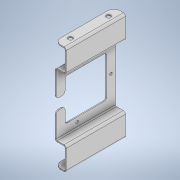
# Autodesk Inventor part: LiDAR_LD19_LD_Plate_1mm_60mmW_Hole
Saved by Autodesk Inventor 2022 (Build 260153000, 153)
## iProperties
Created: 2023-09-22
Part Number: LiDAR_LD19_LD_Plate_1mm_60mmW_Hole
Material: 一般
Document SubType Name: Sheet Metal
Designer: gisen-neige2
Density: 1 g/cm^3
Sheet Metal Rule: Default_mm
Appearance: 既定
Author: gisen-neige2
Autodesk Inventor part; units mm, degrees
ref_plane "YZ Plane" through (0, 0, 0) normal (1, 0, 0) x (0, 1, 0)
ref_plane "XZ Plane" through (0, 0, 0) normal (0, 1, 0) x (-1, 0, 0)
sketch "スケッチ1" plane through (0, 0, 0) normal (0, 1, 0) x (-1, 0, 0)
  line L0 (5.5, 28) -> (-5.5, 28)
  line L1 (-5.5, 28) -> (-5.5, -28)
  line L2 (-5.5, -28) -> (5.5, -28)
  line L3 (5.5, -28) -> (5.5, 28)
  line L4 (5.5, 28) -> (-5.5, -28) construction
  line L5 (-5.5, 28) -> (5.5, -28) construction
  point P0 (0, 0)
  dimension "d0" = 11
  dimension "d1" = 56
  measures "d0" distance of L2.end L1.end
  measures "d1" distance of L1.end L0.end
extrude "プレート1" add sketch "スケッチ1" along normal blind 1
sketch "スケッチ2" plane through (4.5, 1, 28) normal (1, 0, 0) x (0, 1, 0)
  line L0 (0, -56) -> (0, 0)
  line L1 (0, 0) -> (-22, 0)
  line L2 (-22, 0) -> (-22, -56)
  line L3 (-22, -56) -> (0, -56)
  constraints: 6 end point, 1 horizontal, 1 perpendicular, 1 vertical
edge flange "フランジ1" height 22 angle 90 thickness 1 bend radius 1 thickness toward (1, 0, 0) relief tear relief width 1 relief depth 0.5 edges at (5.5, 0, 0) wall of the first edge with corners at (4.5, 1, -28) (4.5, 1, 28) (4.5, -21, 28) (4.5, -21, -28)
bend "曲げ1"
corner "コーナー1"
sketch "スケッチ3" plane through (5.5, -20, 28) normal (0, -1, 0) x (1, 0, 0)
  line L0 (0, -56) -> (0, 0)
  line L1 (0, 0) -> (-10.5, 0)
  line L2 (-10.5, 0) -> (-10.5, -56)
  line L3 (-10.5, -56) -> (0, -56)
  constraints: 6 end point, 1 horizontal, 1 perpendicular, 1 vertical
edge flange "フランジ2" height 10.5 angle 90 thickness 1 bend radius 1 thickness toward (0, -1, 0) relief tear relief width 1 relief depth 0.5 edges at (4.5, -21, 0) wall of the first edge with corners at (5.5, -20, -28) (5.5, -20, 28) (-5, -20, 28) (-5, -20, -28)
bend "曲げ2"
corner "コーナー2"
sketch "スケッチ4" plane through (-4, -20, -28) normal (-1, 0, 0) x (0, -1, 0)
  line L0 (0, 56) -> (0, 0)
  line L1 (0, 0) -> (60, 0)
  line L2 (60, 0) -> (60, 56)
  line L3 (60, 56) -> (0, 56)
  constraints: 6 end point, 1 horizontal, 1 perpendicular, 1 vertical
edge flange "フランジ3" height 60 angle 90 thickness 1 bend radius 1 thickness toward (-1, 0, 0) relief tear relief width 1 relief depth 0.5 edges at (-5, -21, 0) wall of the first edge with corners at (-4, -20, 28) (-4, -20, -28) (-4, -80, -28) (-4, -80, 28)
bend "曲げ3"
corner "コーナー3"
sketch "スケッチ5" plane through (-5, -79, -28) normal (0, -1, 0) x (1, 0, 0)
  line L0 (0, 56) -> (0, 0)
  line L1 (0, 0) -> (10.5, 0)
  line L2 (10.5, 0) -> (10.5, 56)
  line L3 (10.5, 56) -> (0, 56)
  constraints: 6 end point, 1 horizontal, 1 perpendicular, 1 vertical
edge flange "フランジ4" height 10.5 angle 90 thickness 1 bend radius 1 thickness toward (0, -1, 0) relief tear relief width 1 relief depth 0.5 edges at (-4, -80, 0) wall of the first edge with corners at (-5, -79, 28) (-5, -79, -28) (5.5, -79, -28) (5.5, -79, 28)
bend "曲げ4"
corner "コーナー4"
sketch "スケッチ6" plane through (4.5, -79, 28) normal (1, 0, 0) x (0, 1, 0)
  line L0 (0, -56) -> (0, 0)
  line L1 (0, 0) -> (-22, 0)
  line L2 (-22, 0) -> (-22, -56)
  line L3 (-22, -56) -> (0, -56)
  constraints: 6 end point, 1 horizontal, 1 perpendicular, 1 vertical
edge flange "フランジ5" height 22 angle 90 thickness 1 bend radius 1 thickness toward (1, 0, 0) relief tear relief width 1 relief depth 0.5 edges at (5.5, -80, 0) wall of the first edge with corners at (4.5, -79, -28) (4.5, -79, 28) (4.5, -101, 28) (4.5, -101, -28)
bend "曲げ5"
corner "コーナー5"
sketch "スケッチ7" plane through (5.5, -100, 28) normal (0, -1, 0) x (1, 0, 0)
  line L0 (0, -56) -> (0, 0)
  line L1 (0, 0) -> (-11, 0)
  line L2 (-11, 0) -> (-11, -56)
  line L3 (-11, -56) -> (0, -56)
  constraints: 6 end point, 1 horizontal, 1 perpendicular, 1 vertical
edge flange "フランジ6" height 11 angle 90 thickness 1 bend radius 1 thickness toward (0, -1, 0) relief tear relief width 1 relief depth 0.5 edges at (4.5, -101, 0) wall of the first edge with corners at (5.5, -100, -28) (5.5, -100, 28) (-5.5, -100, 28) (-5.5, -100, -28)
bend "曲げ6"
corner "コーナー6"
fillet "コーナーR1" radius 6 4 edges at (-5.5, -100.5, 28) (-5.5, 0.5, -28) (-5.5, 0.5, 28) (-5.5, -100.5, -28)
sketch "スケッチ8" plane through (-4, -22, 28) normal (1, 0, 0) x (0, 0, -1)
  circle A0 centre (19.77, -51.9851) radius 3.6
  circle A1 centre (19.77, -5.1851) radius 3.6
  circle A2 centre (51.69, -28.5851) radius 3.6
  line L0 (9, -47.5851) -> (9, -9.5851)
  circle A3 centre (19.77, -51.9851) radius 2.23
  circle A4 centre (19.77, -5.1851) radius 2.23
  circle A5 centre (51.69, -28.5851) radius 2.23
  line L1 (16.17, -51.9851) -> (16.17, -47.5851)
  line L2 (23.37, -51.9851) -> (23.37, -47.5851)
  line L3 (47, -47.5851) -> (9, -47.5851)
  line L4 (16.17, -5.1851) -> (16.17, -9.5851)
  line L5 (9, -9.5851) -> (47, -9.5851)
  line L6 (23.37, -5.1851) -> (23.37, -9.5851)
  line L7 (51.69, -24.9851) -> (47, -24.9851)
  line L8 (51.69, -32.1851) -> (47, -32.1851)
  line L9 (47, -9.5851) -> (47, -47.5851)
  line L10 (56, -57) -> (0, -57) projected
  line L11 (0, 1) -> (56, 1) projected
  line L12 (56, 0) -> (56, -56) projected
  line L13 (0, -56) -> (56, -56) projected
  point P0 (28, 22)
  point P1 (28, -28)
  dimension "d64" = 7.2
  dimension "d65" = 7.2
  dimension "d66" = 7.2
  dimension "d67" = 46.8
  dimension "d68" = 8.23
  dimension "d69" = 42.69
  dimension "d70" = 23.4
  dimension "d71" = 4.46
  dimension "d72" = 4.46
  dimension "d73" = 4.46
  dimension "d74" = 28
  dimension "d75" = 38
  dimension "d76" = 38
  dimension "d77" = 15.4
  dimension "d78" = 15.4
  dimension "d79" = 23.63
  dimension "d80" = 7.17
  dimension "d81" = 7.17
  dimension "d82" = 23.63
  dimension "d83" = 4.69
  dimension "d84" = 3.6
  dimension "d125" = 28
  dimension "d126" = 18.4149
  constraints: 20 end point, 7 perpendicular, 6 centre point, 6 point on circle, 6 tangent, 4 point on line, 3 coincident
  measures "d64" diameter of A0
  measures "d65" diameter of A1
  measures "d66" diameter of A2
  measures "d67" distance of A1.centre A0.centre
  measures "d68" horizontal distance of point (28, -28) A1.centre
  measures "d69" distance from line of L0 A2.centre
  measures "d70" vertical distance of A0.centre A2.centre
  measures "d71" diameter of A3
  measures "d72" diameter of A4
  measures "d73" diameter of A5
  measures "d74" distance from line of point (28, -28) L12
  measures "d75" distance of L9.end L0.start
  measures "d76" distance of L0.start L5.start
  measures "d77" distance of L7.end L5.end
  measures "d78" distance of L8.end L9.end
  measures "d79" distance of L5.end L6.end
  measures "d80" distance of L5.start L4.end
  measures "d81" distance of L0.start L1.end
  measures "d82" distance of L9.end L2.end
  measures "d83" distance from line of L9 A2.centre
  measures "d84" vertical distance of L8.end A2.centre
  measures "d125" distance from line of L13 point (28, -28)
  measures "d126" distance from line of point (28, -28) L5
hole "穴1" at (-4, -27.1851, 8.23) direction (-1, 0, 0) diameter 2.5 end through all
hole "穴2" at (-4, -73.9851, 8.23) direction (-1, 0, 0) diameter 2.5 end through all
hole "穴3" at (-4, -50.5851, -23.69) direction (-1, 0, 0) diameter 2.5 end through all
ref_plane "作業平面1" through (0, -50, 0) normal (0, 1, 0) x (1, 0, 0)
sketch "スケッチ9" plane through (3.5, -101, -28) normal (0, -1, 0) x (1, 0, 0)
  line L0 (-9, 6) -> (-9, 50) projected
  line L1 (0, 0) -> (-3, 0) projected
  line L2 (-3, 56) -> (0, 56) projected
  point P0 (-3.5, 28)
  point P1 (-4, 46)
  point P2 (-4, 10)
  point P3 (-4, 28)
  dimension "d107" = 5
  dimension "d108" = 5
  dimension "d109" = 10
  dimension "d110" = 10
  dimension "d127" = 56
  dimension "d128" = 28
  constraints: 1 vertical alignment
  measures "d107" distance from line of point (-4, 46) L0
  measures "d108" distance from line of point (-4, 10) L0
  measures "d109" distance from line of point (-4, 10) L1
  measures "d110" distance from line of point (-4, 46) L2
  measures "d127" distance between parallel lines of L2 L1
  measures "d128" distance from line of point (-4, 28) L1
hole "穴4" at (-0.5, -101, 18) at (-0.5, -101, -18) direction (0, 1, 0) diameter 4.2 depth 8 tip angle 118
sketch "スケッチ11" plane through (0, 1, 0) normal (0, 1, 0) x (1, 0, 0)
  point P0 (0, 0)
  point P1 (-0.5, -18)
  point P2 (-0.5, 18)
hole "穴5" at (-0.5, 1, -18) at (-0.5, 1, 18) direction (0, -1, 0) diameter 4.2 depth 1 tip angle 118
hole "穴6" at (-0.5, -101, 0) direction (0, 1, 0) diameter 2 depth 1 tip angle 118
sketch "スケッチ12" plane through (-4, -22, 28) normal (1, 0, 0) x (0, 0, -1)
  line L0 (8.5, -9.0851) -> (47.5, -9.0851)
  line L1 (47.5, -9.0851) -> (47.5, -48.0851)
  line L2 (47.5, -48.0851) -> (8.5, -48.0851)
  line L3 (8.5, -48.0851) -> (8.5, -9.0851)
  line L4 (9, -9.5851) -> (47, -9.5851) projected
  line L5 (47, -47.5851) -> (9, -47.5851) projected
  line L6 (47, -9.5851) -> (47, -47.5851) projected
  line L7 (8.5, -23.5851) -> (0, -23.5851)
  line L8 (0, 0) -> (0, -56) projected
  line L9 (0, -33.5851) -> (8.5, -33.5851)
  circle A0 centre (51.69, -28.5851) radius 1.25 projected
  point P0 (28, 22)
  point P1 (28, -28)
  dimension "d136" = 39
  dimension "d137" = 39
  dimension "d152" = 0.5
  dimension "d153" = 0.5
  dimension "d154" = 5
  dimension "d155" = 5
  constraints: 12 end point, 3 point on line, 2 horizontal, 2 parallel, 2 perpendicular
  measures "d136" distance between parallel lines of L3 L1
  measures "d137" distance between parallel lines of L2 L0
  measures "d152" distance between parallel lines of L4 L0
  measures "d153" distance between parallel lines of L1 L6
  measures "d154" distance from line of A0.centre L7
  measures "d155" distance from line of A0.centre L9
extrude "切り取り4" cut sketch "スケッチ12" against normal blind 1 contours L0 L1 L2 L3
sketch "スケッチ14" plane through (-4, -22, 28) normal (1, 0, 0) x (0, 0, -1)
  line L0 (8.5, -9.0851) -> (8.5, -48.0851) projected
  line L1 (0, 0) -> (0, -56) projected
  line L2 (8.5, -23.5851) -> (0, -23.5851)
  line L3 (0, -23.5851) -> (0, -33.5851)
  line L4 (0, -33.5851) -> (8.5, -33.5851)
  line L5 (8.5, -33.5851) -> (8.5, -23.5851)
  circle A0 centre (51.69, -28.5851) radius 1.25 projected
  point P0 (28, 22)
  dimension "d158" = 10
  dimension "d159" = 5
  constraints: 8 end point, 2 parallel, 2 point on line, 1 horizontal, 1 perpendicular
  measures "d158" distance between parallel lines of L4 L2
  measures "d159" distance from line of A0.centre L4
extrude "切り取り5" cut sketch "スケッチ14" against normal blind 1 contours L0 L4 L1 L2
fillet "コーナーR3" radius 3 4 edges at (-4.5, -45.5851, 28) (-4.5, -55.5851, 28) (-4.5, -45.5851, 19.5) (-4.5, -55.5851, 19.5)
fillet "コーナーR3" radius 2 4 edges at (-4.5, -31.0851, 19.5) (-4.5, -31.0851, -19.5) (-4.5, -70.0851, -19.5) (-4.5, -70.0851, 19.5)
equation "\"d64\" = d66"
equation "\"d65\" = d64"
equation "\"d91\" = Thickness"
equation "\"d123\" = Thickness"
equation "\"d134\" = Thickness"
equation "\"d156\" = Thickness"
equation "\"d159\" = 0.5 * d158"
equation "\"d160\" = Thickness"
equation "\"d2\" = Thickness"
equation "\"d3\" = BendReliefWidth"
equation "\"d4\" = BendReliefDepth"
equation "\"d5\" = MinimumRemnant"
equation "\"d6\" = TransitionRadius"
equation "\"d9\" = BendRadius"
equation "\"d10\" = CornerReliefSize"
equation "\"d11\" = GapSize"
equation "\"d12\" = JacobiRadiusSize"
equation "\"d13\" = BendReliefWidth"
equation "\"d14\" = BendReliefDepth"
equation "\"d15\" = MinimumRemnant"
equation "\"d16\" = TransitionRadius"
equation "\"d19\" = BendRadius"
equation "\"d20\" = CornerReliefSize"
equation "\"d21\" = GapSize"
equation "\"d22\" = JacobiRadiusSize"
equation "\"d23\" = BendReliefWidth"
equation "\"d24\" = BendReliefDepth"
equation "\"d25\" = MinimumRemnant"
equation "\"d26\" = TransitionRadius"
equation "\"d29\" = BendRadius"
equation "\"d30\" = CornerReliefSize"
equation "\"d31\" = GapSize"
equation "\"d32\" = JacobiRadiusSize"
equation "\"d33\" = BendReliefWidth"
equation "\"d34\" = BendReliefDepth"
equation "\"d35\" = MinimumRemnant"
equation "\"d36\" = TransitionRadius"
equation "\"d39\" = BendRadius"
equation "\"d40\" = CornerReliefSize"
equation "\"d41\" = GapSize"
equation "\"d42\" = JacobiRadiusSize"
equation "\"d43\" = BendReliefWidth"
equation "\"d44\" = BendReliefDepth"
equation "\"d45\" = MinimumRemnant"
equation "\"d46\" = TransitionRadius"
equation "\"d49\" = BendRadius"
equation "\"d50\" = CornerReliefSize"
equation "\"d51\" = GapSize"
equation "\"d52\" = JacobiRadiusSize"
equation "\"d53\" = BendReliefWidth"
equation "\"d54\" = BendReliefDepth"
equation "\"d55\" = MinimumRemnant"
equation "\"d56\" = TransitionRadius"
equation "\"d59\" = BendRadius"
equation "\"d60\" = CornerReliefSize"
equation "\"d61\" = GapSize"
equation "\"d62\" = JacobiRadiusSize"
equation "\"d154\" = d155"
equation "\"BendRadius\" = Thickness"
equation "\"BendReliefWidth\" = Thickness"
equation "\"BendReliefDepth\" = 0.5 * Thickness"
equation "\"CornerReliefSize\" = 4 * Thickness"
equation "\"MinimumRemnant\" = 2 * Thickness"
equation "\"TransitionRadius\" = BendRadius"
equation "\"JacobiRadiusSize\" = BendRadius"
equation "\"GapSize\" = Thickness"
equation "\"Thickness\" = 1"
